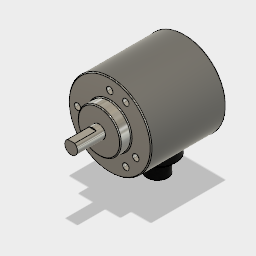
Shaft Encoder 38mm v5 (Autodesk Fusion 360 design; units mm, degrees)
Autodesk Fusion 360 part; units mm, degrees
note: some values were not read from the file. Set by a fixed rule: which sketch regions a step uses.
sketch "Sketch2" plane through (0, 0, 0) normal (0, 0, 1) x (1, 0, 0)
  circle A0 centre (0, 0) radius 19.25
  circle A1 centre (0, 0) radius 10
  circle A2 centre (0, 0) radius 3
  circle A3 centre (0, 0) radius 14 construction
  circle A4 centre (0, 0) radius 15 construction
  line L0 (0, 0) -> (0, 19.25) construction
  circle A5 centre (0, 14) radius 1.5
  circle A6 centre (-12.1244, -7) radius 1.5
  circle A7 centre (12.1244, -7) radius 1.5
  line L1 (0, 0) -> (16.3101, 28.25) construction
  line L2 (0, 0) -> (32.8938, 0) construction
  circle A8 centre (7.5, 12.9904) radius 1.5
  circle A9 centre (-15, 0) radius 1.5
  circle A10 centre (7.5, -12.9904) radius 1.5
  line L3 (-1.6583, 2.5) -> (1.6583, 2.5)
  line L4 (0, 0) -> (0, -32) construction
  line L5 (0, 2.5) -> (0, -3) construction
  dimension "d1" = 38.5
  dimension "d2" = 20
  dimension "d3" = 6
  dimension "d4" = 28
  dimension "d5" = 30
  dimension "d6" = 3
  dimension "d8" = 360
  dimension "d9" = 60
  dimension "d10" = 3
  dimension "d12" = 360
  dimension "d29" = 5.5
  measures "d1" diameter of A0
  measures "d2" diameter of A1
  measures "d3" diameter of A2
  measures "d4" diameter of A3
  measures "d5" diameter of A4
  measures "d6" diameter of A5
  measures "d9" angle of L1 L2
  measures "d10" diameter of A8
  measures "d29" distance of L5.start L5.end
extrude "Extrude1" add sketch "Sketch2" against normal blind 35 contours A0 | A1 | A2 L3 | A2 L3 | A5 | A6 | A7 | A8 | A9 | A10
extrude "Extrude2" cut sketch "Sketch2" against normal blind 8 contours A5 | A6 | A7 | A8 | A9 | A10
extrude "Extrude3" add sketch "Sketch2" along normal blind 5 contours A1 | A2 L3 | A2 L3
extrude "Extrude4" add sketch "Sketch2" along normal blind 18 contours A2 L3 | A2 L3
sketch "Sketch4" plane through (0, 0, 18) normal (0, 0, 1) x (1, 0, 0)
  circle A0 centre (0, 0) radius 3
  line L0 (-1.6583, 2.5) -> (1.6583, 2.5)
  circle A1 centre (0, 0) radius 3
extrude "Extrude5" cut sketch "Sketch4" against normal blind 10 contours A0 L0 A1 picked at (0.41, 2.7801)
fillet "Fillet1" radius 0.4 4 edges at (-9.3233, -3.6162, 5) (-17.9473, -6.9611, 0) (-17.9473, 6.9611, -35) (-9.3233, 3.6162, 0)
sketch "Sketch6" plane through (0, 0, 0) normal (0, 1, 0) x (1, 0, 0)
  line L0 (19.25, 34.6) -> (-19.25, 34.6)
  line L1 (0, 0) -> (0, 44.4198) construction
  circle A0 centre (0, 22.2099) radius 8.5759
  circle A1 centre (0, 22.2099) radius 4.9031
extrude "Extrude6" add sketch "Sketch6" against normal blind 22 contours A0 | A1
extrude "Extrude7" add sketch "Sketch6" against normal blind 30 contours A1
